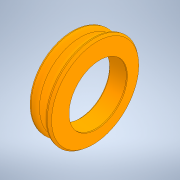
# Autodesk Inventor part: Шкив рычага
Saved by Autodesk Inventor 2021.1 (Build 251245010, 245A)
## iProperties
Created: 2026-05-25
Part Number: Шкив рычага
Material: Типовые
Document SubType Name: Modeling
Designer: Андрей Тарасов
Density: 1 g/cm^3
Appearance: По умолчанию
Author: Андрей Тарасов
Autodesk Inventor part; units mm, degrees
ref_plane "YZ Plane" through (0, 0, 0) normal (1, 0, 0) x (0, 1, 0)
ref_plane "XZ Plane" through (0, 0, 0) normal (0, 1, 0) x (-1, 0, 0)
ref_plane "XY Plane" through (0, 0, 0) normal (0, 0, 1) x (1, 0, 0)
sketch "Эскиз1" plane through (0, 0, 0) normal (0, 0, 1) x (1, 0, 0)
  line L0 (-2.375, 10.1) -> (-1, 10.1)
  line L1 (2.375, 10.1) -> (2.375, 6.6)
  line L2 (2.125, 7) -> (-2.375, 7)
  line L3 (-2.375, 7) -> (-2.375, 10.1)
  line L4 (-3.325, 0) -> (3.325, 0) construction
  line L5 (0, -2.02) -> (0, 12.12) construction
  line L6 (1, 10.1) -> (2.375, 10.1)
  line L7 (-1, 10.1) -> (-0.2, 8.5)
  line L8 (-0.2, 8.5) -> (0.2, 8.5)
  line L9 (0.2, 8.5) -> (1, 10.1)
  line L10 (2.125, 7) -> (2.125, 6.6)
  line L11 (2.125, 6.6) -> (2.375, 6.6)
  point P0 (0, 0)
  point P1 (0, 8.5)
  dimension "d0" = 7
  dimension "d5" = 0.4
  dimension "d6" = 1.5
  dimension "d7" = 2
  dimension "d12" = 0.25
  dimension "d13" = 3.5
  dimension "d14" = 0.4
  dimension "d16" = 4.5
  constraints: 20 end point, 4 perpendicular, 2 equal length, 2 horizontal, 2 point on line, 1 midpoint, 1 vertical
  measures "d0" distance between parallel lines of L2 L4
  measures "d5" distance of L7.end L8.end
  measures "d6" distance between parallel lines of L2 L8
  measures "d7" distance of L6.start L0.end
  measures "d12" distance between parallel lines of L1 L10
  measures "d13" distance of L1.start L1.end
  measures "d14" distance between parallel lines of L2 L11
  measures "d16" distance between parallel lines of L10 L3
revolve "Вращение1" add sketch "Эскиз1" angle 360 about axis through (-10, 0, 0) along (1, 0, 0)
sketch "Эскиз2" plane through (-2.375, 0, 0) normal (-1, 0, 0) x (0, 0, 1)
  circle A0 centre (0, 0) radius 7 construction
  circle A1 centre (0, 7) radius 1
  line L0 (0, -14.14) -> (0, 14.14) construction
  dimension "d21" = 2
  constraints: 1 centre point, 1 point on line, 1 vertical alignment, 1 other
  measures "d21" diameter of A1
extrude "Выдавливание1" cut sketch "Эскиз2" against normal up to surface (4.5 mm away)
fillet "Сопряжение1" radius 1.2 4 edges at (-1, -10.1, 0) (1, -10.1, 0) (-0.125, 6.9286, -0.9974) (-0.125, 6.9286, 0.9974)
chamfer "Фаска2" distance 0.4 angle 45 6 edges at (2.375, -10.1, 0) (-2.375, -10.1, 0) (-2.375, -7, 0) (-2.375, 7.0258, 1.2241) (-2.375, 7.0258, -1.2241) (-2.375, 8, 0)
